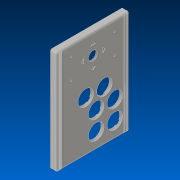
# Autodesk Inventor part: Top
Saved by Autodesk Inventor 2016 (Build 200138000, 138)
## iProperties
Created: 2015-08-21
Part Number: Top
Material: Generic
Document SubType Name: Modeling
Designer: Moffitt
Density: 1 g/cm^3
Appearance: Default
Author: Moffitt
Autodesk Inventor part; units mm, degrees
ref_plane "YZ Plane" through (0, 0, 0) normal (1, 0, 0) x (0, 1, 0)
ref_plane "XZ Plane" through (0, 0, 0) normal (0, 1, 0) x (-1, 0, 0)
ref_plane "XY Plane" through (0, 0, 0) normal (0, 0, 1) x (1, 0, 0)
sketch "Top-Body" plane through (0, 0, 0) normal (1, 0, 0) x (0, 1, 0)
  line L0 (107.2007, 64.0864) -> (-92.7993, 64.0864)
  line L1 (-92.7993, 64.0864) -> (-92.7993, -75.9136)
  line L2 (-92.7993, -75.9136) -> (107.2007, -75.9136)
  line L3 (107.2007, -75.9136) -> (107.2007, 64.0864)
  circle A0 centre (67.2007, -5.9136) radius 9
  circle A1 centre (4.2007, -27.9136) radius 15
  circle A2 centre (-26.2993, -47.9136) radius 15
  circle A3 centre (-62.2993, -47.9136) radius 15
  circle A4 centre (4.2007, 8.0864) radius 15
  circle A5 centre (-26.2993, -11.9136) radius 15
  circle A6 centre (-62.2993, -11.9136) radius 15
  circle A7 centre (87.2007, 36.0864) radius 2.5
  circle A8 centre (87.2007, -47.9136) radius 2.5
  circle A9 centre (47.2007, -47.9136) radius 2.5
  circle A10 centre (47.2007, 36.0864) radius 2.5
  point P0 (0, 0)
  dimension "d0" = 200
  dimension "d1" = 140
  dimension "d2" = 18
  dimension "d3" = 40
  dimension "d5" = 30
  dimension "d6" = 30
  dimension "d7" = 20
  dimension "d8" = 30.5
  dimension "d9" = 30
  dimension "d10" = 36
  dimension "d11" = 0
  dimension "d12" = 63
  dimension "d13" = 30
  dimension "d14" = 30
  dimension "d15" = 30
  dimension "d16" = 36
  dimension "d17" = 36
  dimension "d18" = 36
  dimension "d19" = 0
  dimension "d20" = 0
  dimension "d21" = 0
  dimension "d23" = 14
  dimension "d24" = 70
  dimension "d25" = 5
  dimension "d26" = 42
  dimension "d27" = 20
  dimension "d28" = 20
  dimension "d29" = 20
  dimension "d30" = 20
  dimension "d31" = 42
  dimension "d32" = 42
  dimension "d33" = 70
  dimension "d146" = 42
  dimension "d149" = 5
  dimension "d150" = 5
  dimension "d151" = 5
  constraints: 11 centre point, 8 end point, 2 parallel, 1 horizontal, 1 perpendicular
  measures "d0" distance of L0.start L0.end
  measures "d1" distance of L2.end L0.start
  measures "d2" diameter of A0
  measures "d3" distance from line of L3 A0.centre
  measures "d5" diameter of A1
  measures "d6" diameter of A2
  measures "d7" vertical distance of A2.centre A1.centre
  measures "d8" horizontal distance of A2.centre A1.centre
  measures "d9" diameter of A3
  measures "d10" distance of A3.centre A2.centre
  measures "d11" vertical distance of A3.centre A2.centre
  measures "d12" horizontal distance of A1.centre A0.centre
  measures "d13" diameter of A4
  measures "d14" diameter of A5
  measures "d15" diameter of A6
  measures "d16" distance of A1.centre A4.centre
  measures "d17" distance of A2.centre A5.centre
  measures "d18" distance of A3.centre A6.centre
  measures "d19" horizontal distance of A4.centre A1.centre
  measures "d20" horizontal distance of A5.centre A2.centre
  measures "d21" horizontal distance of A6.centre A3.centre
  measures "d23" vertical distance of A0.centre A4.centre
  measures "d24" distance from line of L2 A0.centre
  measures "d25" diameter of A7
  measures "d26" vertical distance of A0.centre A7.centre
  measures "d27" horizontal distance of A7.centre A0.centre
  measures "d28" horizontal distance of A10.centre A0.centre
  measures "d29" horizontal distance of A0.centre A8.centre
  measures "d30" horizontal distance of A9.centre A0.centre
  measures "d31" vertical distance of A0.centre A8.centre
  measures "d32" vertical distance of A9.centre A0.centre
  measures "d33" distance from line of L0 A0.centre
  measures "d146" vertical distance of A0.centre A10.centre
  measures "d149" diameter of A10
  measures "d150" diameter of A9
  measures "d151" diameter of A8
extrude "Main Face" add sketch "Top-Body" along normal blind 6
fillet "Top Fillet" radius 3 4 edges at (6, 107.2007, -5.9136) (6, 7.2007, 64.0864) (6, 7.2007, -75.9136) (6, -92.7993, -5.9136)
sketch "Button clip cutouts" plane through (0, 0, 0) normal (-1, 0, 0) x (0, 0, 1)
  line L0 (-33.0644, -53.1069) -> (-38.7212, -47.45)
  line L1 (-38.7212, -47.45) -> (-62.7628, -71.4917)
  line L2 (-62.7628, -71.4917) -> (-57.106, -77.1485)
  line L3 (-57.106, -77.1485) -> (-33.0644, -53.1069)
  line L4 (64.0864, -92.7993) -> (-75.9136, -92.7993) projected
  line L5 (2.9356, -71.4917) -> (-2.7212, -77.1485)
  line L6 (-2.7212, -77.1485) -> (-26.7628, -53.1069)
  line L7 (-26.7628, -53.1069) -> (-21.106, -47.45)
  line L8 (-21.106, -47.45) -> (2.9356, -71.4917)
  line L9 (-21.106, -41.1485) -> (-26.7628, -35.4917)
  line L10 (-26.7628, -35.4917) -> (-2.7212, -11.45)
  line L11 (-2.7212, -11.45) -> (2.9356, -17.1069)
  line L12 (2.9356, -17.1069) -> (-21.106, -41.1485)
  line L13 (-38.7212, -41.1485) -> (-33.0644, -35.4917)
  line L14 (-33.0644, -35.4917) -> (-57.106, -11.45)
  line L15 (-57.106, -11.45) -> (-62.7628, -17.1069)
  line L16 (-62.7628, -17.1069) -> (-38.7212, -41.1485)
  circle A0 centre (-47.9136, -26.2993) radius 15 projected
  circle A1 centre (-11.9136, -26.2993) radius 15 projected
  line L17 (-1.106, -10.6485) -> (-6.7628, -4.9917)
  line L18 (-6.7628, -4.9917) -> (17.2788, 19.05)
  line L19 (17.2788, 19.05) -> (22.9356, 13.3931)
  line L20 (22.9356, 13.3931) -> (-1.106, -10.6485)
  line L21 (-23.9136, -12.7993) -> (-31.9136, -12.7993)
  line L22 (-31.9136, -12.7993) -> (-31.9136, 21.2007)
  line L23 (-31.9136, 21.2007) -> (-23.9136, 21.2007)
  line L24 (-23.9136, 21.2007) -> (-23.9136, -12.7993)
  circle A2 centre (8.0864, 4.2007) radius 15 projected
  circle A3 centre (-27.9136, 4.2007) radius 15 projected
  point P0 (0, 0)
  point P1 (-11.9136, -62.2993)
  point P2 (-47.9136, -62.2993)
  dimension "d46" = 45
  dimension "d48" = 17
  dimension "d49" = 4
  dimension "d50" = 4
  dimension "d52" = 4
  dimension "d53" = 4
  dimension "d54" = 17
  dimension "d55" = 17
  dimension "d56" = 17
  dimension "d57" = 90
  dimension "d58" = 90
  dimension "d59" = 90
  dimension "d60" = 90
  dimension "d61" = 90
  dimension "d62" = 90
  dimension "d63" = 34
  dimension "d64" = 8
  dimension "d65" = 8
  dimension "d66" = 4
  dimension "d67" = 17
  dimension "d68" = 34
  dimension "d69" = 8
  dimension "d70" = 90
  dimension "d73" = 17
  dimension "d74" = 4
  dimension "d77" = 135
  dimension "d78" = 90
  dimension "d79" = 90
  dimension "d81" = 90
  dimension "d82" = 90
  dimension "d83" = 90
  dimension "d85" = 90
  dimension "d86" = 90
  dimension "d87" = 90
  dimension "d88" = 34
  dimension "d89" = 8
  dimension "d90" = 4
  dimension "d91" = 17
  dimension "d92" = 90
  dimension "d93" = 90
  dimension "d94" = 34
  dimension "d95" = 17
  dimension "d96" = 4
  dimension "d97" = 8
  constraints: 48 end point, 10 perpendicular, 1 horizontal, 1 parallel, 1 point on line
  measures "d46" angle of L4 L3
  measures "d48" distance from line of L0 point (-47.914, -62.299)
  measures "d49" distance from line of L1 point (-47.914, -62.299)
  measures "d50" distance from line of L3 point (-47.914, -62.299)
  measures "d52" distance from line of L8 point (-11.914, -62.299)
  measures "d53" distance from line of L6 point (-11.914, -62.299)
  measures "d54" distance from line of L5 point (-11.914, -62.299)
  measures "d55" distance from line of L7 point (-11.914, -62.299)
  measures "d56" distance from line of L2 point (-47.914, -62.299)
  measures "d57" angle of L10 L9
  measures "d58" angle of L11 L12
  measures "d59" angle of L9 L12
  measures "d60" angle of L10 L11
  measures "d61" angle of L16 L13
  measures "d62" angle of L15 L14
  measures "d63" distance between parallel lines of L15 L13
  measures "d64" distance of L13.start L13.end
  measures "d65" distance of L14.end L15.end
  measures "d66" distance from line of L14 A0.centre
  measures "d67" distance from line of L13 A0.centre
  measures "d68" distance of L9.end L10.end
  measures "d69" distance of L9.start L9.end
  measures "d70" angle of L14 L10
  measures "d73" distance from line of A1.centre L11
  measures "d74" distance from line of L10 A1.centre
  measures "d77" angle of L4 L8
  measures "d78" angle of L5 L8
  measures "d79" angle of L6 L7
  measures "d81" angle of L8 L12
  measures "d82" angle of L6 L3
  measures "d83" angle of L16 L1
  measures "d85" angle of L17 L20
  measures "d86" angle of L20 L19
  measures "d87" angle of L17 L10
  measures "d88" distance of L19.end L17.start
  measures "d89" distance of L18.end L19.end
  measures "d90" distance from line of L20 A2.centre
  measures "d91" distance from line of L17 A2.centre
  measures "d92" angle of L21 L24
  measures "d93" angle of L23 L22
  measures "d94" distance of L21.end L22.end
  measures "d95" distance from line of L21 A3.centre
  measures "d96" distance from line of L22 A3.centre
  measures "d97" distance of L22.end L23.end
extrude "Button Snap Cutouts" cut sketch "Button clip cutouts" against normal blind 3 contours L3 L2 L1 L0 | L5 L6 L7 L8 | L9 L10 A1 L12 | A1 L10 L12 | A1 L10 L11 L12 | L16 A0 L14 L13 | L16 A0 L14 | L16 L15 L14 A0 | L17 L18 A2 L20 | A2 L18 L20 | A2 L18 L19 L20 | L21 L22 A3 L24 | A3 L22 L24 | A3 L22 L23 L24
chamfer "Button Snap Chamfers" distance 0.5 angle 45 48 edges at (1.5, -69.6934, -60.9645) (1.5, -49.2483, -40.5195) (1.5, -54.9052, -34.8626) (1.5, -54.9052, -24.9645) (1.5, -49.2483, -19.3077) (1.5, -75.3502, -4.5195) (1.5, -69.6934, 1.1374) (1.5, -75.3502, -55.3077) (1.5, -77.1485, -57.106) (1.5, -71.4917, -62.7628) (1.5, -47.45, -38.7212) (1.5, -53.1069, -33.0644) (1.5, -53.1069, -26.7628) (1.5, -47.45, -21.106) (1.5, -71.4917, 2.9356) (1.5, -77.1485, -2.7212) (1.5, -39.3502, -40.5195) (1.5, -41.1485, -38.7212) (1.5, -35.4917, -33.0644) (1.5, -33.6934, -34.8626) (1.5, -13.2483, -55.3077) (1.5, -11.45, -57.106) (1.5, -18.9052, -60.9645) (1.5, -17.1069, -62.7628) (1.5, -35.4917, -26.7628) (1.5, -41.1485, -21.106) (1.5, -39.3502, -19.3077) (1.5, -33.6934, -24.9645) (1.5, -13.2483, -4.5195) (1.5, -11.45, -2.7212) (1.5, -17.1069, 2.9356) (1.5, -18.9052, 1.1374) (1.5, -10.2561, -23.9136) (1.5, -12.7993, -23.9136) (1.5, -12.7993, -31.9136) (1.5, -10.2561, -31.9136) (1.5, 18.6576, -31.9136) (1.5, 21.2007, -31.9136) (1.5, 21.2007, -23.9136) (1.5, 18.6576, -23.9136) (1.5, -3.1934, -4.9645) (1.5, -4.9917, -6.7628) (1.5, -10.6485, -1.106) (1.5, -8.8502, 0.6923) (1.5, 17.2517, 15.4805) (1.5, 19.05, 17.2788) (1.5, 13.3931, 22.9356) (1.5, 11.5948, 21.1374)
sketch "sweet lines" plane through (0, -92.7993, -75.9136) normal (0, -1, 0) x (1, 0, 0)
  line L0 (6, 137) -> (6, 3) projected
  line L1 (6, 4.5) -> (4.5, 4.5)
  line L2 (4.5, 4.5) -> (4.5, 6.5)
  line L3 (4.5, 6.5) -> (6, 6.5)
  line L4 (6, 6.5) -> (6, 4.5)
  line L5 (6, 8.5) -> (4.5, 8.5)
  line L6 (4.5, 8.5) -> (4.5, 10.5)
  line L7 (4.5, 10.5) -> (6, 10.5)
  line L8 (6, 10.5) -> (6, 8.5)
  line L9 (6, 135.5) -> (4.5, 135.5)
  line L10 (4.5, 135.5) -> (4.5, 133.5)
  line L11 (4.5, 133.5) -> (6, 133.5)
  line L12 (6, 133.5) -> (6, 135.5)
  line L13 (6, 132) -> (4.5, 132)
  line L14 (4.5, 132) -> (4.5, 130)
  line L15 (4.5, 130) -> (6, 130)
  line L16 (6, 130) -> (6, 132)
  point P0 (0, 75.9136)
  dimension "d103" = 2
  dimension "d104" = 1.5
  dimension "d105" = 2
  dimension "d106" = 2
  dimension "d107" = 1.5
  dimension "d110" = 1.5
  dimension "d111" = 2
  dimension "d112" = 2
  dimension "d113" = 1.5
  dimension "d114" = 1.5
  dimension "d115" = 1.5
  dimension "d116" = 1.5
  constraints: 32 end point, 8 parallel, 5 point on line, 4 horizontal, 4 perpendicular
  measures "d103" distance of L1.end L2.end
  measures "d104" distance of L1.start L1.end
  measures "d105" distance between parallel lines of L5 L3
  measures "d106" distance of L5.end L6.end
  measures "d107" distance of L5.start L5.end
  measures "d110" distance from line of L0.end L1
  measures "d111" distance of L13.end L14.end
  measures "d112" distance of L9.end L10.end
  measures "d113" distance from line of L9 L0.start
  measures "d114" distance between parallel lines of L13 L11
  measures "d115" distance of L14.end L15.end
  measures "d116" distance of L10.end L11.end
extrude "SNOW WHITE DESIGN PATTERNS" cut sketch "sweet lines" against normal blind 200
sketch "Insignias" plane through (6, 0, 0) normal (1, 0, 0) x (0, 0, -1)
  line L0 (24.9136, 72.2007) -> (24.9136, 62.2007)
  line L1 (24.9136, 62.2007) -> (29.9136, 67.2007)
  line L2 (29.9136, 67.2007) -> (24.9136, 72.2007)
  circle A0 centre (5.9136, 67.2007) radius 9 projected
  line L3 (10.9136, 48.2007) -> (0.9136, 48.2007)
  line L4 (0.9136, 48.2007) -> (5.9136, 43.2007)
  line L5 (5.9136, 43.2007) -> (10.9136, 48.2007)
  line L6 (10.9136, 85.2007) -> (0.9136, 85.2007)
  line L7 (0.9136, 85.2007) -> (5.9136, 90.2007)
  line L8 (5.9136, 90.2007) -> (10.9136, 85.2007)
  line L9 (-12.0864, 62.2007) -> (-12.0864, 72.2007)
  line L10 (-12.0864, 72.2007) -> (-17.0864, 67.2007)
  line L11 (-17.0864, 67.2007) -> (-12.0864, 62.2007)
  point P0 (0, 0)
  dimension "d117" = 45
  dimension "d118" = 45
  dimension "d119" = 10
  dimension "d120" = 10
  dimension "d121" = 5
  dimension "d122" = 45
  dimension "d123" = 45
  dimension "d124" = 10
  dimension "d125" = 10
  dimension "d126" = 5
  dimension "d127" = 19
  dimension "d128" = 18
  dimension "d129" = 18
  constraints: 24 end point, 3 perpendicular, 2 horizontal, 2 point on line, 1 vertical
  measures "d117" angle of L0 L2
  measures "d118" angle of L0 L1
  measures "d119" distance of L0.start L0.end
  measures "d120" distance edge to line of A0 L0
  measures "d121" vertical distance of A0.centre L0.start
  measures "d122" angle of L5 L3
  measures "d123" angle of L3 L4
  measures "d124" distance of L3.start L3.end
  measures "d125" distance edge to line of A0 L3
  measures "d126" horizontal distance of L3.end A0.centre
  measures "d127" distance from line of A0.centre L0
  measures "d128" distance from line of A0.centre L6
  measures "d129" distance from line of L9 A0.centre
extrude "Insignias Extrusion" cut sketch "Insignias" against normal blind 1.5 contours L2 L1 L0 | L5 L4 L3 | L6 L7 L8 | L11 L10 L9
sketch "Border" plane through (0, 0, 0) normal (-1, 0, 0) x (0, 0, 1)
  line L0 (-71.9136, -88.7993) -> (60.0864, -88.7993)
  line L1 (60.0864, -88.7993) -> (60.0864, 103.2007)
  line L2 (60.0864, 103.2007) -> (-71.9136, 103.2007)
  line L3 (-71.9136, 103.2007) -> (-71.9136, -88.7993)
  line L4 (64.0864, -92.7993) -> (-75.9136, -92.7993) projected
  line L5 (-75.9136, 107.2007) -> (64.0864, 107.2007) projected
  line L6 (-75.9136, -92.7993) -> (-75.9136, 107.2007) projected
  line L7 (64.0864, 107.2007) -> (64.0864, -92.7993) projected
  point P0 (0, 0)
  dimension "d132" = 4
  dimension "d133" = 4
  dimension "d134" = 4
  dimension "d135" = 4
  constraints: 8 end point, 2 parallel, 1 horizontal, 1 perpendicular
  measures "d132" distance between parallel lines of L4 L0
  measures "d133" distance between parallel lines of L5 L2
  measures "d134" distance between parallel lines of L6 L3
  measures "d135" distance between parallel lines of L7 L1
extrude "Walls" add sketch "Border" along normal blind 6
fillet "Fillet3" radius 3 8 edges at (5.1213, 106.322, 63.2077) (-1.5, 107.2007, 64.0864) (5.1213, 106.322, -75.0349) (-1.5, 107.2007, -75.9136) (5.1213, -91.9206, 63.2077) (-1.5, -92.7993, 64.0864) (5.1213, -91.9206, -75.0349) (-1.5, -92.7993, -75.9136)
sketch "Connection Lip" plane through (-6, 0, 0) normal (-1, 0, 0) x (0, 0, 1)
  line L0 (-72.4136, -91.2993) -> (60.5864, -91.2993)
  line L1 (62.5864, -89.2993) -> (62.5864, 103.7007)
  line L2 (60.5864, 105.7007) -> (-72.4136, 105.7007)
  line L3 (-74.4136, 103.7007) -> (-74.4136, -89.2993)
  line L4 (-72.9136, -92.7993) -> (61.0864, -92.7993) projected
  line L5 (-75.9136, 104.2007) -> (-75.9136, -89.7993) projected
  line L6 (61.0864, 107.2007) -> (-72.9136, 107.2007) projected
  line L7 (64.0864, -89.7993) -> (64.0864, 104.2007) projected
  arc A0 (-74.4136, -89.2993) -> (-72.4136, -91.2993) centre (-72.4136, -89.2993) ccw
  arc A1 (-72.4136, 105.7007) -> (-74.4136, 103.7007) centre (-72.4136, 103.7007) ccw
  arc A2 (62.5864, 103.7007) -> (60.5864, 105.7007) centre (60.5864, 103.7007) ccw
  arc A3 (60.5864, -91.2993) -> (62.5864, -89.2993) centre (60.5864, -89.2993) ccw
  point P0 (0, 0)
  dimension "d139" = 1.5
  dimension "d140" = 1.5
  dimension "d141" = 1.5
  dimension "d142" = 1.5
  dimension "d143" = 2
  constraints: 8 end point, 8 point on circle, 8 tangent, 4 centre point, 3 equal radius, 2 parallel, 1 horizontal, 1 perpendicular
  measures "d139" distance between parallel lines of L4 L0
  measures "d140" distance between parallel lines of L5 L3
  measures "d141" distance between parallel lines of L6 L2
  measures "d142" distance between parallel lines of L7 L1
  measures "d143" radius of A0
extrude "Extrusion6" cut sketch "Connection Lip" against normal blind 3
sketch "Sketch10" plane through (0, 0, 0) normal (-1, 0, 0) x (0, 0, 1)
  line L0 (-51.9136, 93.7007) -> (40.0864, 93.7007)
  line L1 (42.0864, 91.7007) -> (42.0864, 42.7007)
  line L2 (40.0864, 40.7007) -> (-51.9136, 40.7007)
  line L3 (-53.9136, 42.7007) -> (-53.9136, 91.7007)
  circle A0 centre (-47.9136, 87.2007) radius 2.5 projected
  circle A1 centre (-5.9136, 67.2007) radius 9 projected
  circle A2 centre (-47.9136, 47.2007) radius 2.5 projected
  arc A3 (-51.9136, 93.7007) -> (-53.9136, 91.7007) centre (-51.9136, 91.7007) ccw
  arc A4 (-53.9136, 42.7007) -> (-51.9136, 40.7007) centre (-51.9136, 42.7007) ccw
  arc A5 (40.0864, 40.7007) -> (42.0864, 42.7007) centre (40.0864, 42.7007) ccw
  arc A6 (42.0864, 91.7007) -> (40.0864, 93.7007) centre (40.0864, 91.7007) ccw
  point P0 (0, 0)
  point P1 (-53.9136, 93.7007)
  point P2 (42.0864, 93.7007)
  dimension "d155" = 96
  dimension "d157" = 48
  dimension "d158" = 6.5
  dimension "d159" = 6.5
  dimension "d160" = 2
  constraints: 8 end point, 8 point on circle, 8 tangent, 4 centre point, 4 point on line, 3 equal radius, 2 parallel, 1 horizontal, 1 perpendicular
  measures "d155" distance of point (-53.914, 93.701) point (42.086, 93.701)
  measures "d157" distance from line of L3 A1.centre
  measures "d158" vertical distance of point (-53.914, 93.701) A0.centre
  measures "d159" distance from line of L2 A2.centre
  measures "d160" radius of A3
extrude "Extrusion7" cut sketch "Sketch10" against normal blind 2
sketch "Sketch11" plane through (0, 0, 0) normal (-1, 0, 0) x (0, 0, 1)
  line L0 (53.0864, 77.2007) -> (52.0864, 77.2007)
  line L1 (52.0864, 77.2007) -> (52.0864, 76.2007)
  line L2 (52.0864, 76.2007) -> (49.0864, 76.2007)
  line L3 (49.0864, 76.2007) -> (49.0864, 77.2007)
  line L4 (49.0864, 77.2007) -> (50.0864, 77.2007)
  line L5 (50.0864, 77.2007) -> (50.0864, 78.2007)
  line L6 (50.0864, 78.2007) -> (48.0864, 78.2007)
  line L7 (48.0864, 78.2007) -> (48.0864, 75.2007)
  line L8 (48.0864, 75.2007) -> (52.0864, 75.2007)
  line L9 (52.0864, 75.2007) -> (52.0864, 74.2007)
  line L10 (52.0864, 74.2007) -> (53.0864, 74.2007)
  line L11 (53.0864, 74.2007) -> (53.0864, 77.2007)
  line L12 (53.0864, 73.2007) -> (48.0864, 73.2007)
  line L13 (48.0864, 73.2007) -> (48.0864, 69.2007)
  line L14 (48.0864, 69.2007) -> (49.0864, 69.2007)
  line L15 (49.0864, 69.2007) -> (49.0864, 72.2007)
  line L16 (49.0864, 72.2007) -> (53.0864, 72.2007)
  line L17 (53.0864, 72.2007) -> (53.0864, 73.2007)
  line L18 (42.0864, 91.7007) -> (42.0864, 42.7007) projected
  line L19 (53.0864, 68.2007) -> (53.0864, 65.2007)
  line L20 (53.0864, 65.2007) -> (52.0864, 65.2007)
  line L21 (52.0864, 65.2007) -> (52.0864, 67.2007)
  line L22 (52.0864, 67.2007) -> (51.0864, 67.2007)
  line L23 (51.0864, 67.2007) -> (51.0864, 66.2007)
  line L24 (51.0864, 66.2007) -> (50.0864, 66.2007)
  line L25 (50.0864, 66.2007) -> (50.0864, 67.2007)
  line L26 (53.0864, 68.2007) -> (48.0864, 68.2007)
  line L27 (48.0864, 68.2007) -> (48.0864, 67.2007)
  line L28 (48.0864, 67.2007) -> (50.0864, 67.2007)
  line L29 (51.0864, 64.2007) -> (50.0864, 64.2007)
  line L30 (50.0864, 64.2007) -> (50.0864, 62.2007)
  line L31 (50.0864, 62.2007) -> (51.0864, 62.2007)
  line L32 (51.0864, 62.2007) -> (51.0864, 64.2007)
  line L33 (48.0864, 61.2007) -> (53.0864, 61.2007)
  line L34 (53.0864, 61.2007) -> (53.0864, 59.2007)
  line L35 (53.0864, 59.2007) -> (52.0864, 59.2007)
  line L36 (52.0864, 59.2007) -> (52.0864, 60.2007)
  line L37 (52.0864, 60.2007) -> (51.0864, 60.2007)
  line L38 (51.0864, 60.2007) -> (51.0864, 59.2007)
  line L39 (51.0864, 59.2007) -> (50.0864, 59.2007)
  line L40 (50.0864, 59.2007) -> (50.0864, 60.2007)
  line L41 (50.0864, 60.2007) -> (48.0864, 60.2007)
  line L42 (48.0864, 60.2007) -> (48.0864, 61.2007)
  line L43 (52.0864, 59.2007) -> (51.0864, 59.2007)
  line L44 (51.0864, 58.2007) -> (52.0864, 58.2007)
  line L45 (52.0864, 58.2007) -> (52.0864, 59.2007)
  line L46 (51.0864, 59.2007) -> (51.0864, 58.2007)
  line L47 (52.0864, 57.2007) -> (51.0864, 57.2007)
  line L48 (51.0864, 57.2007) -> (51.0864, 56.2007)
  line L49 (51.0864, 56.2007) -> (52.0864, 56.2007)
  line L50 (52.0864, 56.2007) -> (52.0864, 57.2007)
  line L51 (53.0864, 56.2007) -> (48.0864, 56.2007)
  line L52 (48.0864, 56.2007) -> (48.0864, 55.2007)
  line L53 (48.0864, 55.2007) -> (53.0864, 55.2007)
  line L54 (53.0864, 55.2007) -> (53.0864, 56.2007)
  line L55 (18.0864, -47.7993) -> (13.0864, -47.7993)
  line L56 (13.0864, -47.7993) -> (13.0864, -49.7993)
  line L57 (13.0864, -49.7993) -> (14.0864, -49.7993)
  line L58 (14.0864, -49.7993) -> (14.0864, -50.7993)
  line L59 (14.0864, -50.7993) -> (15.0864, -50.7993)
  line L60 (15.0864, -50.7993) -> (15.0864, -49.7993)
  line L61 (15.0864, -49.7993) -> (16.0864, -49.7993)
  line L62 (16.0864, -49.7993) -> (16.0864, -50.7993)
  line L63 (16.0864, -50.7993) -> (17.0864, -50.7993)
  line L64 (17.0864, -50.7993) -> (17.0864, -49.7993)
  line L65 (17.0864, -49.7993) -> (18.0864, -49.7993)
  line L66 (18.0864, -49.7993) -> (18.0864, -47.7993)
  line L67 (17.0864, -49.7993) -> (16.0864, -49.7993)
  line L68 (16.0864, -49.7993) -> (16.0864, -48.7993)
  line L69 (16.0864, -48.7993) -> (17.0864, -48.7993)
  line L70 (17.0864, -48.7993) -> (17.0864, -49.7993)
  line L71 (15.0864, -49.7993) -> (14.0864, -49.7993)
  line L72 (14.0864, -49.7993) -> (14.0864, -48.7993)
  line L73 (14.0864, -48.7993) -> (15.0864, -48.7993)
  line L74 (15.0864, -48.7993) -> (15.0864, -49.7993)
  line L75 (14.0864, -51.7993) -> (13.0864, -51.7993)
  line L76 (13.0864, -51.7993) -> (13.0864, -54.7993)
  line L77 (13.0864, -54.7993) -> (14.0864, -54.7993)
  line L78 (14.0864, -54.7993) -> (16.0864, -54.7993)
  line L79 (16.0864, -54.7993) -> (16.0864, -52.7993)
  line L80 (16.0864, -52.7993) -> (17.0864, -52.7993)
  line L81 (17.0864, -52.7993) -> (17.0864, -54.7993)
  line L82 (17.0864, -54.7993) -> (18.0864, -54.7993)
  line L83 (18.0864, -54.7993) -> (18.0864, -51.7993)
  line L84 (18.0864, -51.7993) -> (15.0864, -51.7993)
  line L85 (15.0864, -51.7993) -> (15.0864, -53.7993)
  line L86 (15.0864, -53.7993) -> (14.0864, -53.7993)
  line L87 (14.0864, -53.7993) -> (14.0864, -51.7993)
  line L88 (13.0864, -55.7993) -> (18.0864, -55.7993)
  line L89 (18.0864, -55.7993) -> (18.0864, -58.7993)
  line L90 (18.0864, -58.7993) -> (17.0864, -58.7993)
  line L91 (17.0864, -58.7993) -> (17.0864, -56.7993)
  line L92 (17.0864, -56.7993) -> (16.0864, -56.7993)
  line L93 (16.0864, -56.7993) -> (16.0864, -57.7993)
  line L94 (16.0864, -57.7993) -> (15.0864, -57.7993)
  line L95 (15.0864, -57.7993) -> (15.0864, -56.7993)
  line L96 (15.0864, -56.7993) -> (13.0864, -56.7993)
  line L97 (13.0864, -56.7993) -> (13.0864, -55.7993)
  line L98 (60.0864, 103.2007) -> (-71.9136, 103.2007) projected
  arc A0 (-18.8686, -39.5894) -> (1.3765, -19.3443) centre (-11.9136, -26.2993) ccw projected
  line L99 (-71.9136, -88.7993) -> (60.0864, -88.7993) projected
  line L100 (18.0864, -46.7993) -> (13.0864, -46.7993)
  line L101 (13.0864, -46.7993) -> (13.0864, -43.7993)
  line L102 (13.0864, -43.7993) -> (18.0864, -43.7993)
  line L103 (18.0864, -43.7993) -> (18.0864, -46.7993)
  line L104 (17.0864, -44.7993) -> (14.0864, -44.7993)
  line L105 (14.0864, -44.7993) -> (14.0864, -45.7993)
  line L106 (14.0864, -45.7993) -> (17.0864, -45.7993)
  line L107 (17.0864, -45.7993) -> (17.0864, -44.7993)
  point P0 (0, 0)
  dimension "d163" = 1
  dimension "d164" = 3
  dimension "d165" = 2
  dimension "d166" = 1
  dimension "d167" = 1
  dimension "d168" = 3
  dimension "d169" = 1
  dimension "d170" = 1
  dimension "d171" = 1
  dimension "d172" = 3
  dimension "d173" = 1
  dimension "d177" = 1
  dimension "d178" = 1
  dimension "d179" = 1
  dimension "d182" = 3
  dimension "d183" = 1
  dimension "d185" = 6
  dimension "d186" = 0
  dimension "d187" = 2
  dimension "d188" = 1
  dimension "d189" = 1
  dimension "d190" = 1
  dimension "d191" = 1
  dimension "d192" = 2
  dimension "d193" = 1
  dimension "d194" = 5
  dimension "d195" = 1
  dimension "d196" = 1
  dimension "d197" = 1
  dimension "d198" = 5
  dimension "d211" = 2
  dimension "d212" = 1
  dimension "d214" = 1
  dimension "d215" = 1
  dimension "d216" = 3
  dimension "d217" = 3
  dimension "d218" = 1
  dimension "d219" = 1
  dimension "d220" = 1
  dimension "d221" = 1
  dimension "d222" = 25
  dimension "d227" = 30
  dimension "d228" = 1
  dimension "d231" = 3
  dimension "d232" = 1
  dimension "d233" = 1
  dimension "d234" = 1
  dimension "d235" = 1
  constraints: 210 end point, 65 perpendicular, 41 point on line, 12 horizontal, 9 parallel, 1 vertical
  measures "d163" distance of L0.start L0.end
  measures "d164" distance of L1.end L2.end
  measures "d165" distance of L5.end L6.end
  measures "d166" distance of L16.end L12.start
  measures "d167" distance between parallel lines of L2 L8
  measures "d168" distance of L10.end L0.start
  measures "d169" distance of L2.end L3.end
  measures "d170" distance of L4.end L5.end
  measures "d171" distance between parallel lines of L10 L12
  measures "d172" distance of L14.end L15.end
  measures "d173" distance of L13.end L14.end
  measures "d177" distance of L19.end L20.end
  measures "d178" distance of L21.end L22.end
  measures "d179" distance of L23.end L24.end
  measures "d182" distance of L19.start L19.end
  measures "d183" distance of L22.end L23.end
  measures "d185" distance between parallel lines of L18 L7
  measures "d186" distance between parallel lines of L19 L17
  measures "d187" distance of L31.end L29.start
  measures "d188" distance between parallel lines of L29 L20
  measures "d189" distance between parallel lines of L14 L26
  measures "d190" distance between parallel lines of L33 L31
  measures "d191" distance between parallel lines of L37 L33
  measures "d192" distance of L33.end L34.end
  measures "d193" distance of L38.end L44.start
  measures "d194" distance of L33.start L33.end
  measures "d195" distance of L49.end L47.start
  measures "d196" distance of L53.end L51.start
  measures "d197" distance between parallel lines of L44 L47
  measures "d198" distance of L52.end L53.end
  measures "d211" distance of L65.end L55.start
  measures "d212" distance of L63.end L64.end
  measures "d214" distance between parallel lines of L84 L63
  measures "d215" distance between parallel lines of L88 L82
  measures "d216" distance of L82.end L83.end
  measures "d217" distance of L88.end L89.end
  measures "d218" distance of L94.end L95.end
  measures "d219" distance of L96.end L88.start
  measures "d220" distance between parallel lines of L84 L80
  measures "d221" distance between parallel lines of L78 L86
  measures "d222" distance between parallel lines of L98 L6
  measures "d227" distance between parallel lines of L99 L90
  measures "d228" distance of L69.end L64.end
  measures "d231" distance of L102.end L100.start
  measures "d232" distance between parallel lines of L55 L100
  measures "d233" distance between parallel lines of L100 L106
  measures "d234" distance between parallel lines of L102 L104
  measures "d235" distance of L26.end L27.end
extrude "Extrusion10" cut sketch "Sketch11" against normal blind 3 contours L11 L10 L9 L8 L7 L6 L5 L4 L3 L2 L1 L0 | L17 L16 L15 L14 L13 L12 | L19 L20 L21 L22 L23 L24 L25 L28 L27 L26 | L32 L31 L30 L29 | L33 L34 L35 L36 L37 L38 L39 L40 L41 L42 | L45 L44 L46 L43 | L50 L49 L48 L47 | L51 L54 L53 L52 L49 | L66 L65 L70 L69 L68 L61 L74 L73 L72 L57 L56 L55 | L64 L63 L62 L67 | L71 L60 L59 L58 | L87 L86 L85 L84 L83 L82 L81 L80 L79 L78 L77 L76 L75 | L88 L89 L90 L91 L92 L93 L94 L95 L96 L97 | L100 L101 L102 L103
body "Solid1"
